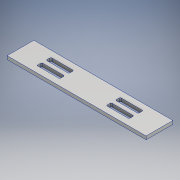
# Autodesk Inventor part: BK-BKT120-Front
Saved by Autodesk Inventor 2017 (Build 210142000, 142)
## iProperties
Created: 2016-09-24
Part Number: BK-BKT120-Front
Material: Aluminum 6061
Document SubType Name: Modeling
Designer: vslabsal
Density: 2.7 g/cm^3
Appearance: Aluminum - Flat
Author: vslabsal
Autodesk Inventor part; units mm, degrees
ref_plane "YZ Plane" through (0, 0, 0) normal (1, 0, 0) x (0, 1, 0)
ref_plane "XZ Plane" through (0, 0, 0) normal (0, 1, 0) x (-1, 0, 0)
ref_plane "XY Plane" through (0, 0, 0) normal (0, 0, 1) x (1, 0, 0)
sketch "Sketch1" plane through (0, 0, 0) normal (0, 0, 1) x (1, 0, 0)
  line L0 (-197.485, -38.1) -> (197.485, -38.1)
  line L1 (197.485, -38.1) -> (197.485, 38.1)
  line L2 (197.485, 38.1) -> (-197.485, 38.1)
  line L3 (-197.485, 38.1) -> (-197.485, -38.1)
  line L4 (-197.485, -38.1) -> (197.485, 38.1) construction
  line L5 (197.485, -38.1) -> (-197.485, 38.1) construction
  line L6 (66, -6) -> (131, -20) construction
  line L7 (131, -6) -> (66, -20) construction
  arc A0 (69.175, -6) -> (66, -9.175) centre (69.175, -9.175) ccw
  arc A1 (66, -16.825) -> (69.175, -20) centre (69.175, -16.825) ccw
  arc A2 (127.825, -20) -> (131, -16.825) centre (127.825, -16.825) ccw
  arc A3 (131, -9.175) -> (127.825, -6) centre (127.825, -9.175) ccw
  line L8 (66, -9.175) -> (66, -16.825)
  line L9 (69.175, -20) -> (127.825, -20)
  line L10 (131, -16.825) -> (131, -9.175)
  line L11 (69.175, -6) -> (127.825, -6)
  line L12 (66, 20) -> (131, 6) construction
  line L13 (131, 20) -> (66, 6) construction
  arc A4 (69.175, 20) -> (66, 16.825) centre (69.175, 16.825) ccw
  arc A5 (66, 9.175) -> (69.175, 6) centre (69.175, 9.175) ccw
  arc A6 (127.825, 6) -> (131, 9.175) centre (127.825, 9.175) ccw
  arc A7 (131, 16.825) -> (127.825, 20) centre (127.825, 16.825) ccw
  line L14 (66, 16.825) -> (66, 9.175)
  line L15 (69.175, 6) -> (127.825, 6)
  line L16 (131, 9.175) -> (131, 16.825)
  line L17 (69.175, 20) -> (127.825, 20)
  line L18 (-131, -6) -> (-66, -20) construction
  line L19 (-66, -6) -> (-131, -20) construction
  arc A8 (-127.825, -6) -> (-131, -9.175) centre (-127.825, -9.175) ccw
  arc A9 (-131, -16.825) -> (-127.825, -20) centre (-127.825, -16.825) ccw
  arc A10 (-69.175, -20) -> (-66, -16.825) centre (-69.175, -16.825) ccw
  arc A11 (-66, -9.175) -> (-69.175, -6) centre (-69.175, -9.175) ccw
  line L20 (-131, -9.175) -> (-131, -16.825)
  line L21 (-127.825, -20) -> (-69.175, -20)
  line L22 (-66, -16.825) -> (-66, -9.175)
  line L23 (-127.825, -6) -> (-69.175, -6)
  arc A12 (-66, 16.825) -> (-69.175, 20) centre (-69.175, 16.825) ccw
  line L24 (-127.825, 20) -> (-69.175, 20)
  line L25 (-127.825, 6) -> (-69.175, 6)
  line L26 (-131, 20) -> (-66, 6) construction
  line L27 (-66, 20) -> (-131, 6) construction
  line L28 (-131, 16.825) -> (-131, 9.175)
  arc A13 (-127.825, 20) -> (-131, 16.825) centre (-127.825, 16.825) ccw
  arc A14 (-131, 9.175) -> (-127.825, 6) centre (-127.825, 9.175) ccw
  line L29 (-66, 9.175) -> (-66, 16.825)
  arc A15 (-69.175, 6) -> (-66, 9.175) centre (-69.175, 9.175) ccw
  point P0 (0, 0)
  point P1 (0, 0)
  point P2 (98.5, -13)
  point P3 (98.5, 13)
  point P4 (-98.5, -13)
  point P5 (-98.5, 13)
  dimension "d0" = 394.97
  dimension "d1" = 76.2
  constraints: 60 end point, 40 point on circle, 16 centre point, 12 point on line, 10 midpoint, 9 horizontal, 8 vertical, 2 parallel, 1 perpendicular
  measures "d0" distance of L0.start L0.end
  measures "d1" distance of L0.end L1.end
extrude "Extrusion2" add sketch "Sketch1" along normal blind 9.525
body "Solid2"
